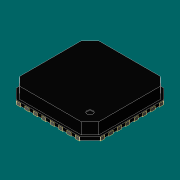
# Autodesk Inventor part: qfn-32
Saved by Autodesk Inventor 2016 (Build 200138000, 138)
## iProperties
Created: 2015-10-12
Part Number: qfn-32
Material: ABS Plastic
Document SubType Name: Modeling
Designer: Sawaiz
Density: 1.06 g/cm^3
Appearance: Smooth - Black
width: 5.000 mm
length: 5.000 mm
height: 0.900 mm
leadFrame: 0.200 mm
seatingHeight: 0.050 mm
padSpacing: 0.500 mm
padDepth: 0.500 mm
padWidth: 0.250 mm
numLeads: 32.000 ul
Author: Sawaiz
Autodesk Inventor part; units mm, degrees
ref_plane "YZ Plane" through (0, 0, 0) normal (1, 0, 0) x (0, 1, 0)
ref_plane "XZ Plane" through (0, 0, 0) normal (0, 1, 0) x (-1, 0, 0)
ref_plane "XY Plane" through (0, 0, 0) normal (0, 0, 1) x (1, 0, 0)
sketch "Sketch1" plane through (0, 0, 0) normal (0, 0, 1) x (1, 0, 0)
  line L0 (2.5, -2.5) -> (-2.5, -2.5)
  line L1 (-2.5, -2.5) -> (-2.5, 2.5)
  line L2 (-2.5, 2.5) -> (2.5, 2.5)
  line L3 (2.5, 2.5) -> (2.5, -2.5)
  line L4 (2.5, -2.5) -> (-2.5, 2.5) construction
  line L5 (-2.5, -2.5) -> (2.5, 2.5) construction
  point P0 (0, 0)
  dimension "d0" = 5
  dimension "d1" = 5
  constraints: 12 end point, 2 midpoint, 2 parallel, 1 horizontal, 1 perpendicular
  measures "d0" distance of L1.end L2.end
  measures "d1" distance of L0.end L1.end
extrude "Extrusion1" add sketch "Sketch1" along normal blind 0.85
sketch "Sketch2" plane through (0, 0, 0) normal (0, 0, -1) x (-1, 0, 0)
  line L0 (-2.5, -2.5) -> (2.5, -2.5) projected
  line L1 (2.5, -2.5) -> (2.5, 2.5) projected
  line L2 (2.5, 2.5) -> (-2.5, 2.5) projected
  line L3 (-2.5, 2.5) -> (-2.5, -2.5) projected
  circle A0 centre (-2.125, 0.25) radius 0.125
  line L4 (-2.125, 0.375) -> (-2.5, 0.375)
  line L5 (-2.125, 0.125) -> (-2.5, 0.125)
  line L6 (-2.5, -2.5) -> (-2.5, 2.5) projected
  point P0 (0, 0)
  point P1 (-2.5, 0)
  dimension "d4" = 0.25
  dimension "d5" = 0.375
  dimension "d66" = 0.25
  constraints: 4 end point, 2 point on circle, 2 point on line, 2 tangent, 1 centre point, 1 midpoint, 1 parallel, 1 perpendicular
  measures "d4" diameter of A0
  measures "d5" distance from line of L3 A0.centre
  measures "d66" vertical distance of A0.centre point (-2.5, 0)
extrude "Extrusion2" cut sketch "Sketch2" against normal blind 0.15 contours L3 L4 A0 L5 | A0
sketch "Sketch3" plane through (0, 0, 0) normal (0, 0, -1) x (-1, 0, 0)
  line L0 (-1.5, -1.5) -> (1.5, -1.5)
  line L1 (1.5, -1.5) -> (1.5, 1.5)
  line L2 (1.5, 1.5) -> (-1.05, 1.5)
  line L3 (-1.5, 1.05) -> (-1.5, -1.5)
  line L4 (-1.5, -1.5) -> (1.5, 1.5) construction
  line L5 (1.5, -1.5) -> (-1.5, 1.5) construction
  line L6 (-1.05, 1.5) -> (-1.5, 1.05)
  point P0 (0, 0)
  dimension "d14" = 3
  dimension "d15" = 3
  dimension "d16" = 0.45
  dimension "d17" = 0.45
  constraints: 14 end point, 2 midpoint, 2 parallel, 2 point on line, 1 horizontal, 1 perpendicular
  measures "d14" distance of L5.end L1.end
  measures "d15" distance of L1.end L0.end
  measures "d16" distance of L2.end L5.end
  measures "d17" distance of L3.start L5.end
extrude "Extrusion3" add sketch "Sketch3" along normal blind 0.05
sketch "Sketch5" plane through (0, 0, 0.85) normal (0, 0, 1) x (1, 0, 0)
  circle A0 centre (1.6, 1.6) radius 0.18
  line L0 (2.5, -2.5) -> (2.5, 2.5) projected
  line L1 (2.5, 2.5) -> (-2.5, 2.5) projected
  point P0 (0, 0)
  dimension "d29" = 0.36
  dimension "d30" = 0.9
  dimension "d31" = 0.9
  constraints: 1 centre point
  measures "d29" diameter of A0
  measures "d30" distance from line of L0 A0.centre
  measures "d31" distance from line of L1 A0.centre
extrude "Extrusion5" cut sketch "Sketch5" against normal blind 0.05
pattern_linear "Rectangular Pattern3" count 8 spacing 0.5 along (0, -1, 0) of "Extrusion2" first direction both ways yes
mirror "Mirror1" about plane through (0, 0, 0) normal (1, 0, 0) of "Extrusion2", "Rectangular Pattern3"
sketch "Sketch6" plane through (0, 0, 0) normal (0, 0, -1) x (-1, 0, 0)
  line L0 (2.5, 2.5) -> (-2.5, 2.5) projected
  circle A0 centre (0.25, 2.125) radius 0.125
  line L1 (0.125, 2.125) -> (0.125, 2.5)
  line L2 (0.375, 2.125) -> (0.375, 2.5)
  line L3 (-2.5, 2.5) -> (2.5, 2.5) projected
  point P0 (0, 0)
  point P1 (0, 2.5)
  dimension "d37" = 0.25
  dimension "d38" = 0.375
  dimension "d67" = 0.25
  constraints: 4 end point, 2 point on circle, 2 point on line, 2 tangent, 1 centre point, 1 midpoint, 1 perpendicular, 1 vertical
  measures "d37" diameter of A0
  measures "d38" distance from line of L0 A0.centre
  measures "d67" horizontal distance of A0.centre point (0, 2.5)
extrude "Extrusion6" cut sketch "Sketch6" against normal blind 0.15
pattern_linear "Rectangular Pattern4" count 8 spacing 0.5 along (1, 0, 0) of "Extrusion6" first direction both ways yes
mirror "Mirror2" about plane through (0, 0, 0) normal (0, 1, 0) of "Extrusion6", "Rectangular Pattern4"
sketch "Sketch7" plane through (0, 0, 0.15) normal (0, 0, -1) x (-1, 0, 0)
  line L0 (-2.125, 0.125) -> (-2.5, 0.125) projected
  arc A0 (-2.125, 0.125) -> (-2.125, 0.375) centre (-2.125, 0.25) ccw projected
  line L1 (-2.5, 0.375) -> (-2.125, 0.375) projected
  line L2 (-2.5, 0.125) -> (-2.5, 0.375) projected
  point P0 (0, 0)
extrude "Extrusion7" add sketch "Sketch7" along normal blind 0.2 separate body
pattern_linear "Rectangular Pattern5" count 8 spacing 0.5 along (0, -1, 0) of "Extrusion7" first direction both ways yes bodies 2
mirror "Mirror4" about plane through (0, 0, 0) normal (1, 0, 0) of "Extrusion7", "Rectangular Pattern5" bodies 2
sketch "Sketch9" plane through (0, 0, 0.15) normal (0, 0, -1) x (-1, 0, 0)
  arc A0 (0.125, 2.125) -> (0.375, 2.125) centre (0.25, 2.125) ccw projected
  line L0 (0.375, 2.5) -> (0.375, 2.125) projected
  line L1 (0.125, 2.5) -> (0.375, 2.5) projected
  line L2 (0.125, 2.125) -> (0.125, 2.5) projected
  point P0 (0, 0)
extrude "Extrusion9" add sketch "Sketch9" along normal blind 0.2 separate body
pattern_linear "Rectangular Pattern7" count 8 spacing 0.5 along (1, 0, 0) of "Extrusion9" first direction both ways yes bodies 3
mirror "Mirror3" about plane through (0, 0, 0) normal (0, 1, 0) of "Extrusion9", "Rectangular Pattern7" bodies 3
chamfer "Chamfer1" distance 0.6 angle 45 4 edges at (2.5, 2.5, 0.425) (-2.5, 2.5, 0.425) (-2.5, -2.5, 0.425) (2.5, -2.5, 0.425)
sketch "Sketch11" plane through (0, 0, 0.85) normal (0, 0, 1) x (1, 0, 0)
  circle A0 centre (1.6, 1.6) radius 0.18 projected
  line L0 (-1.9, -2.5) -> (1.9, -2.5) projected
  line L1 (2.5, -1.9) -> (2.5, 1.9) projected
  line L2 (1.9, 2.5) -> (-1.9, 2.5) projected
  line L3 (-2.5, 1.9) -> (-2.5, -1.9) projected
  line L4 (2.5, -1.9) -> (1.9, -2.5) projected
  line L5 (1.9, 2.5) -> (2.5, 1.9) projected
  line L6 (-2.5, 1.9) -> (-1.9, 2.5) projected
  line L7 (-1.9, -2.5) -> (-2.5, -1.9) projected
  line L8 (1.8482, -2.375) -> (-1.8482, -2.375)
  line L9 (-1.8482, -2.375) -> (-2.375, -1.8482)
  line L10 (-2.375, -1.8482) -> (-2.375, 1.8482)
  line L11 (-2.375, 1.8482) -> (-1.8482, 2.375)
  line L12 (-1.8482, 2.375) -> (1.8482, 2.375)
  line L13 (1.8482, 2.375) -> (2.375, 1.8482)
  line L14 (2.375, 1.8482) -> (2.375, -1.8482)
  line L15 (2.375, -1.8482) -> (1.8482, -2.375)
  point P0 (0, 0)
  dimension "d78" = 0.125
  constraints: 16 end point, 7 other
  measures "d78" distance between parallel lines of L0 L8
extrude "Extrusion11" cut sketch "Sketch11" against normal blind 0.65 contours L7 L3 L6 L2 L5 L1 L4 L0 bodies 1
draft "FaceDraft1" angle 2.5 pull direction (0, 0, 1) fixed plane through (2.4583, 0.6161, 0.2) normal (0, 0, 1) faces at (2.375, 0.6161, 0.6333) (2.0238, 2.1994, 0.6333) (-0.6161, 2.375, 0.6333) (-2.1994, 2.0238, 0.6333) (-2.375, -0.6161, 0.6333) (-2.0238, -2.1994, 0.6333) (0.6161, -2.375, 0.6333) (2.1994, -2.0238, 0.6333)
equation "\"d0\" = width"
equation "\"d1\" = length"
equation "\"d2\" = height - seatingHeight"
equation "\"d4\" = padWidth"
equation "\"d5\" = padDepth - 0.5 * padWidth"
equation "\"d6\" = leadFrame - seatingHeight"
equation "\"d14\" = 0.6 * width"
equation "\"d15\" = 0.6 * length"
equation "\"d16\" = 0.5 * height"
equation "\"d17\" = d16"
equation "\"d18\" = seatingHeight"
equation "\"d29\" = 0.4 * height"
equation "\"d30\" = height"
equation "\"d31\" = height"
equation "\"d32\" = seatingHeight"
equation "\"d36\" = padSpacing"
equation "\"d37\" = padWidth"
equation "\"d38\" = padDepth - 0.5 * padWidth"
equation "\"d39\" = leadFrame - seatingHeight"
equation "\"d43\" = padSpacing"
equation "\"d44\" = leadFrame"
equation "\"d48\" = padSpacing"
equation "\"d54\" = leadFrame"
equation "\"d58\" = padSpacing"
equation "\"width\" = 5"
equation "\"length\" = 5"
equation "\"height\" = 0.9"
equation "\"leadFrame\" = 0.2"
equation "\"seatingHeight\" = 0.05"
equation "\"padSpacing\" = 0.5"
equation "\"padDepth\" = 0.5"
equation "\"padWidth\" = 0.25"
equation "\"numLeads\" = 32"
body "Solid1"
body "Solid2"
body "Solid4"
